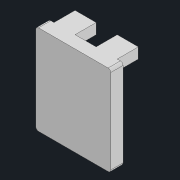
# Autodesk Inventor part: base_link
Saved by Autodesk Inventor 2021 (Build 250183000, 183)
## iProperties
Created: 2021-07-10
Part Number: base_link
Material: 一般
Document SubType Name: Modeling
Designer: yuta0
Density: 1 g/cm^3
Appearance: 既定
Author: yuta0
Autodesk Inventor part; units mm, degrees
ref_plane "YZ Plane" through (0, 0, 0) normal (1, 0, 0) x (0, 1, 0)
ref_plane "XZ Plane" through (0, 0, 0) normal (0, 1, 0) x (-1, 0, 0)
ref_plane "XY Plane" through (0, 0, 0) normal (0, 0, 1) x (1, 0, 0)
sketch "スケッチ1" plane through (0, 0, 0) normal (0, 0, 1) x (1, 0, 0)
  line L0 (-71, -85) -> (71, -85)
  line L1 (71, -85) -> (71, 85)
  line L2 (71, 85) -> (-71, 85)
  line L3 (-71, 85) -> (-71, -85)
  line L4 (-71, -85) -> (71, 85) construction
  line L5 (71, -85) -> (-71, 85) construction
  point P0 (0, 0)
  dimension "d0" = 142
  dimension "d1" = 170
  constraints: 12 end point, 2 midpoint, 2 parallel, 1 horizontal, 1 perpendicular
  measures "d0" distance of L1.end L2.end
  measures "d1" distance of L0.end L1.end
extrude "押し出し1" add sketch "スケッチ1" along normal blind 23.35
fillet "フィレット1" radius 5 4 edges at (-71, 85, 11.675) (-71, -85, 11.675) (71, 85, 11.675) (71, -85, 11.675)
sketch "スケッチ2" plane through (0, 0, 0) normal (0, 0, 1) x (1, 0, 0)
  arc A0 (66, -85) -> (71, -80) centre (66, -80) ccw projected
  line L0 (71, -80) -> (71, 80) projected
  arc A1 (71, 80) -> (66, 85) centre (66, 80) ccw projected
  line L1 (66, 85) -> (-66, 85) projected
  arc A2 (-66, 85) -> (-71, 80) centre (-66, 80) ccw projected
  line L2 (-71, 80) -> (-71, -80) projected
  arc A3 (-71, -80) -> (-66, -85) centre (-66, -80) ccw projected
  line L3 (-66, -85) -> (66, -85) projected
  line L4 (-60, 65) -> (60, 65)
  line L5 (60, 65) -> (60, 85)
  line L6 (60, 85) -> (-60, 85)
  line L7 (-60, 85) -> (-60, 65)
  line L8 (-60, 65) -> (60, 85) construction
  line L9 (60, 65) -> (-60, 85) construction
  line L10 (66, 85) -> (-66, 85) projected
  line L11 (-20, 85) -> (-20, 65)
  line L12 (20, 65) -> (20, 85)
  point P0 (0, 0)
  point P1 (0, 75)
  point P2 (0, 75)
  dimension "d5" = 120
  dimension "d6" = 20
  dimension "d9" = 40
  dimension "d10" = 40
  constraints: 16 end point, 5 point on line, 3 midpoint, 3 perpendicular, 2 parallel, 1 horizontal, 1 vertical alignment
  measures "d5" distance of L5.end L6.end
  measures "d6" distance of L6.end L4.start
  measures "d9" distance between parallel lines of L7 L11
  measures "d10" distance between parallel lines of L5 L12
extrude "押し出し2" add sketch "スケッチ2" against normal blind 40 contours L5 L4 L12 L1 | L1 L11 L4 L7
